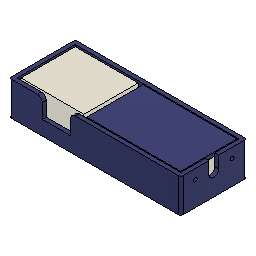
Breadboard Box Fusion (Autodesk Fusion 360 design; units mm, degrees)
Autodesk Fusion 360 part; units mm, degrees
sketch "Sketch1" plane through (0, 0, 0) normal (0, 1, 0) x (1, 0, 0)
  line L0 (0, 0) -> (165, 0)
  line L1 (165, 0) -> (165, -56)
  line L2 (165, -56) -> (0, -56)
  line L3 (0, -56) -> (0, 0)
  dimension "d1" = 165
  dimension "d2" = 56
  constraint horizontal L0
  constraint vertical L1
  constraint horizontal L2
  constraint vertical L3
  constraint coincident L0.start L3.end
  measures "d1" distance of L0.start L0.end
  measures "d2" distance of L0.start L2.end
extrude "Extrude1" add sketch "Sketch1" along normal blind 10 makes body 1
sketch "Sketch2" plane through (0, 10, 0) normal (0, 1, 0) x (-1, 0, 0)
  line L0 (0, 56) -> (-165, 56)
  line L1 (-165, 56) -> (-165, 0)
  line L2 (-165, 0) -> (0, 0)
  line L3 (0, 0) -> (0, 56)
  line L4 (0, 0) -> (-65, 0)
  line L5 (-65, 0) -> (-65, 56)
  line L6 (-65, 56) -> (0, 56)
  line L7 (0, 56) -> (0, 0)
  line L8 (-165, 15) -> (-115, 15)
  line L9 (-115, 15) -> (-115, 41)
  line L10 (-115, 41) -> (-165, 41)
  line L11 (-165, 41) -> (-165, 15)
  dimension "d5" = 65
  dimension "d8" = 15
  dimension "d9" = 15
  dimension "d10" = 50
  constraint horizontal L4
  constraint vertical L5
  constraint horizontal L6
  constraint vertical L7
  constraint coincident L2.end L3.start
  constraint horizontal L8
  constraint vertical L9
  constraint horizontal L10
  constraint vertical L11
  constraint coincident L1 L8.start
  measures "d5" distance of L2.end L4.end
  measures "d8" distance of L1.end L8.start
  measures "d9" distance of L0.end L10.end
  measures "d10" distance of L9 L11
extrude "Extrude2" add sketch "Sketch2" along normal blind 20 contours L0 L2 L3 L4 L5 L6 L7 bodies 1
extrude "Extrude3" add sketch "Sketch2" along normal blind 15 contours L1 L8 L9 L10 L11 bodies 1
sketch "Sketch3" plane through (0, 0, 0) normal (0, -1, 0) x (1, 0, 0)
  line L0 (165, 56) -> (0, 56)
  line L1 (0, 56) -> (0, 0)
  line L2 (0, 0) -> (165, 0)
  line L3 (165, 0) -> (165, 56)
  line L4 (-2, -2) -> (167, -2)
  line L5 (167, -2) -> (167, 58)
  line L6 (167, 58) -> (-2, 58)
  line L7 (-2, 58) -> (-2, -2)
  line L8 (-6, -6) -> (171, -6)
  line L9 (171, -6) -> (171, 62)
  line L10 (171, 62) -> (-6, 62)
  line L11 (-6, 62) -> (-6, -6)
  dimension "d13" = 2
  dimension "d14" = 6
extrude "Extrude4" add sketch "Sketch3" along normal blind 5 separate body contours L0 L1 L2 L3 | L4 L5 L6 L7 | L8 L9 L10 L11 makes body 2
extrude "Extrude5" add sketch "Sketch3" against normal blind 30 contours L8 L9 L10 L11 bodies 2
sketch "Sketch5" plane through (171, 0, 0) normal (1, 0, 0) x (0, 0, -1)
  line L0 (-62, 30) -> (-62, -5)
  line L1 (-62, -5) -> (6, -5)
  line L2 (6, -5) -> (6, 30)
  line L3 (6, 30) -> (-62, 30)
  line L4 (-28, 30) -> (-28, -5)
  line L5 (-28, 30) -> (-28, 17.5)
  arc A0 (-33, 17.5) -> (-23, 17.5) centre (-28, 17.5) ccw
  line L6 (-33, 17.5) -> (-33, 30)
  line L7 (-23, 17.5) -> (-23, 30)
  dimension "d19" = 12.5
  dimension "d20" = 5
  constraint midpoint L3 L4.start
  constraint midpoint L1 L4.end
  constraint perpendicular L3 L5
  constraint coincident L5.end A0.centre
  constraint coincident L3 L6.end
  constraint tangent A0 L6
  constraint perpendicular L3 L6
  constraint coincident L3 L7.end
  constraint tangent A0 L7
  constraint perpendicular L3 L7
  measures "d19" distance of L4.start L5.end
  measures "d20" radius of A0
extrude "Extrude6" cut sketch "Sketch5" against normal blind 4 contours L3 L4 L5 A0 L6 | L3 L4 L5 A0 L7 bodies 2
sketch "Sketch6" plane through (0, 30, 0) normal (0, 1, 0) x (-1, 0, 0)
  line L0 (-171, 33) -> (-167, 33)
  line L1 (-167, 33) -> (-167, 58)
  line L2 (-167, 58) -> (2, 58)
  line L3 (2, 58) -> (2, -2)
  line L4 (2, -2) -> (-167, -2)
  line L5 (-167, -2) -> (-167, 23)
  line L6 (-167, 23) -> (-171, 23)
  line L7 (-171, 23) -> (-171, -6)
  line L8 (-171, -6) -> (6, -6)
  line L9 (6, -6) -> (6, 62)
  line L10 (6, 62) -> (-171, 62)
  line L11 (-171, 62) -> (-171, 33)
  line L12 (0, 56) -> (-65, 56)
  line L13 (-65, 56) -> (-65, 0)
  line L14 (-65, 0) -> (0, 0)
  line L15 (0, 0) -> (0, 56)
  line L16 (-68, -2) -> (-68, 58)
  line L17 (-68, 58) -> (-167, 58)
  line L18 (-167, 58) -> (-167, -2)
  line L19 (-167, -2) -> (-68, -2)
  line L20 (-68, -2) -> (-68, 58)
  line L21 (-69, 57) -> (-166, 57)
  line L22 (-166, 57) -> (-166, -1)
  line L23 (-166, -1) -> (-69, -1)
  line L24 (-69, -1) -> (-69, 57)
  dimension "d23" = 3
  dimension "d35" = -1
  constraint coincident L4 L16.start
  constraint coincident L2 L16.end
  constraint perpendicular L2 L16
  constraint horizontal L17
  constraint vertical L18
  constraint horizontal L19
  constraint vertical L20
  constraint coincident L4.end L5.start
  measures "d23" distance of L13 L16
extrude "Extrude7" add sketch "Sketch6" against normal blind 4 separate body contours L21 L22 L23 L24 makes body 3
sketch "Sketch7" plane through (0, 0, -2) normal (0, 0, 1) x (1, 0, 0)
  line L0 (-2, 0) -> (167, 0)
  line L1 (167, 0) -> (167, 30)
  line L2 (167, 30) -> (-2, 30)
  line L3 (-2, 30) -> (-2, 0)
  line L4 (82.5, 30) -> (87.5, 30)
  line L5 (87.5, 30) -> (87.5, 18)
  line L6 (87.5, 18) -> (82.5, 18)
  line L7 (82.5, 18) -> (82.5, 30)
  line L8 (142.5, 30) -> (147.5, 30)
  line L9 (147.5, 30) -> (147.5, 18)
  line L10 (147.5, 18) -> (142.5, 18)
  line L11 (142.5, 18) -> (142.5, 30)
  line L12 (82.5, 28) -> (87.5, 28)
  line L13 (142.5, 28) -> (147.5, 28)
  dimension "d26" = 5
  dimension "d27" = 12
  dimension "d28" = 5
  dimension "d29" = 12
  dimension "d30" = 55
  dimension "d34" = 2
  constraint horizontal L4
  constraint vertical L5
  constraint horizontal L6
  constraint vertical L7
  constraint midpoint L2 L4.start
  constraint horizontal L8
  constraint vertical L9
  constraint horizontal L10
  constraint vertical L11
  constraint coincident L2 L8.start
  constraint coincident L7 L12.start
  constraint coincident L5 L12.end
  constraint perpendicular L5 L12
  constraint coincident L11 L13.start
  constraint coincident L9 L13.end
  constraint perpendicular L9 L13
  constraint collinear L12 L13
  measures "d26" distance of L4.start L4.end
  measures "d27" distance of L4.start L6.end
  measures "d28" distance of L8.start L8.end
  measures "d29" distance of L8.start L10.end
  measures "d30" distance of L5 L8.start
  measures "d34" distance of L4 L12
revolve "Revolve1" cut sketch "Sketch7" angle 10 about axis through (142.5, 28, -2) along (1, 0, 0) contours L5 L6 L7 L12 | L9 L10 L11 L13 bodies 2
ref_plane "WorkPlane1" through (82.5, 15, 28) normal (0, 0, 1) x (1, 0, 0)
mirror "Mirror1" about plane through (82.5, 15, 28) normal (0, 0, 1) of "Revolve1"
sketch "Sketch8" plane through (0, 26, 0) normal (0, -1, 0) x (1, 0, 0)
  line L0 (69, 57) -> (69, -1)
  line L1 (69, -1) -> (166, -1)
  line L2 (166, -1) -> (166, 57)
  line L3 (166, 57) -> (69, 57)
  line L4 (82.5, 58) -> (87.5, 58)
  line L5 (87.5, 58) -> (82.5, 58)
  line L6 (142.5, 58) -> (147.5, 58)
  line L7 (147.5, 58) -> (142.5, 58)
  line L8 (167, 58) -> (-2, 58)
  line L9 (-2, 58) -> (167, 58)
  line L10 (87.5, -2) -> (82.5, -2)
  line L11 (82.5, -2) -> (87.5, -2)
  line L12 (147.5, -2) -> (142.5, -2)
  line L13 (142.5, -2) -> (147.5, -2)
  line L14 (-2, -2) -> (167, -2)
  line L15 (167, -2) -> (-2, -2)
  line L16 (147.5, -1) -> (142.5, -1)
  line L17 (142.5, -1) -> (142.5, 2)
  line L18 (142.5, 2) -> (147.5, 2)
  line L19 (147.5, 2) -> (147.5, -1)
  line L20 (166, 28) -> (69, 28)
  line L21 (87.5, -1) -> (82.5, -1)
  line L22 (82.5, -1) -> (82.5, 2)
  line L23 (82.5, 2) -> (87.5, 2)
  line L24 (87.5, 2) -> (87.5, -1)
  line L25 (82.5, 54) -> (87.5, 54)
  line L26 (82.5, 57) -> (82.5, 54)
  line L27 (87.5, 54) -> (87.5, 57)
  line L28 (147.5, 54) -> (147.5, 57)
  line L29 (142.5, 54) -> (147.5, 54)
  line L30 (142.5, 57) -> (142.5, 54)
  dimension "d36" = 3
  dimension "d37" = 3
  constraint horizontal L16
  constraint vertical L17
  constraint horizontal L18
  constraint vertical L19
  constraint coincident L1 L16.start
  constraint midpoint L2 L20.start
  constraint midpoint L0 L20.end
  constraint horizontal L21
  constraint vertical L22
  constraint horizontal L23
  constraint vertical L24
  constraint coincident L1 L21.start
  constraint collinear L10.end L21.end L22.end
  constraint vertical L10.start L21.start
  constraint vertical L12.end L16.end
  constraint vertical L12.start L16.start
  constraint symmetric L16.start L20 L28.end
  constraint symmetric L16.end L20 L30.start
  constraint symmetric L17.end L20 L29.start
  constraint symmetric L18.end L20 L28.start
  constraint symmetric L20 L21.start L27.end
  constraint symmetric L20 L21.end L26.start
  constraint symmetric L20 L22.end L25.start
  constraint symmetric L20 L23.end L25.end
  measures "d36" distance of L16.start L18.end
  measures "d37" distance of L21.start L23.end
extrude "Extrude8" add sketch "Sketch8" along normal blind 7.5 contours L3 L25 L26 L27 | L1 L21 L22 L23 L24 | L3 L28 L29 L30 | L1 L16 L17 L18 L19 bodies 3
sketch "Sketch9" plane through (0, 0, 57) normal (0, 0, 1) x (1, 0, 0)
  line L0 (166, 30) -> (69, 30)
  line L1 (69, 30) -> (69, 26)
  line L2 (69, 26) -> (82.5, 26)
  line L3 (82.5, 26) -> (82.5, 18.5)
  line L4 (82.5, 18.5) -> (87.5, 18.5)
  line L5 (87.5, 18.5) -> (87.5, 26)
  line L6 (87.5, 26) -> (142.5, 26)
  line L7 (142.5, 26) -> (142.5, 18.5)
  line L8 (142.5, 18.5) -> (147.5, 18.5)
  line L9 (147.5, 18.5) -> (147.5, 26)
  line L10 (147.5, 26) -> (166, 26)
  line L11 (166, 26) -> (166, 30)
  line L12 (82.5, 26) -> (87.5, 26)
  line L13 (87.5, 26) -> (87.5, 18.5)
  line L14 (87.5, 18.5) -> (82.5, 18.5)
  line L15 (82.5, 18.5) -> (82.5, 26)
  line L16 (142.5, 18.5) -> (147.5, 18.5)
  line L17 (147.5, 18.5) -> (147.5, 26)
  line L18 (147.5, 26) -> (142.5, 26)
  line L19 (142.5, 26) -> (142.5, 18.5)
  constraint horizontal L12
  constraint vertical L13
  constraint horizontal L14
  constraint vertical L15
  constraint coincident L4.end L5.start
  constraint coincident L2.end L3.start
  constraint horizontal L16
  constraint vertical L17
  constraint horizontal L18
  constraint vertical L19
  constraint coincident L9.end L10.start
  constraint coincident L7.end L8.start
revolve "Revolve2" add sketch "Sketch9" angle 15 about axis through (82.5, 26, 57) along (-1, 0, 0) contours L7 L8 L9 L16 L17 L18 L19 | L3 L4 L5 L12 L13 L14 L15 bodies 3
sketch "Sketch10" plane through (0, 0, -1) normal (0, 0, -1) x (-1, 0, 0)
  line L0 (-69, 30) -> (-166, 30)
  line L1 (-166, 30) -> (-166, 26)
  line L2 (-166, 26) -> (-147.5, 26)
  line L3 (-147.5, 26) -> (-147.5, 18.5)
  line L4 (-147.5, 18.5) -> (-142.5, 18.5)
  line L5 (-142.5, 18.5) -> (-142.5, 26)
  line L6 (-142.5, 26) -> (-87.5, 26)
  line L7 (-87.5, 26) -> (-87.5, 18.5)
  line L8 (-87.5, 18.5) -> (-82.5, 18.5)
  line L9 (-82.5, 18.5) -> (-82.5, 26)
  line L10 (-82.5, 26) -> (-69, 26)
  line L11 (-69, 26) -> (-69, 30)
  line L12 (-87.5, 26) -> (-82.5, 26)
  line L13 (-142.5, 26) -> (-147.5, 26)
  constraint coincident L6.end L7.start
  constraint coincident L9.end L10.start
  constraint coincident L5.end L6.start
  constraint coincident L2.end L3.start
revolve "Revolve3" add sketch "Sketch10" angle 15 about axis through (87.5, 26, -1) along (1, 0, 0) contours L7 L8 L9 L12 | L3 L4 L5 L13 bodies 3
fillet "Fillet1" radius 1.5 4 edges at (145, 18.7556, 58.9411) (85, 18.7556, 58.9411) (85, 18.7556, -2.9411) (145, 18.7556, -2.9411) on bodies 3
sketch "Sketch11" plane through (171, 0, 0) normal (1, 0, 0) x (0, 0, -1)
  line L0 (-33, 17.5) -> (-33, 30)
  line L1 (-33, 30) -> (-62, 30)
  line L2 (-62, 30) -> (-62, -5)
  line L3 (-62, -5) -> (6, -5)
  line L4 (6, -5) -> (6, 30)
  line L5 (6, 30) -> (-23, 30)
  line L6 (-23, 30) -> (-23, 17.5)
  arc A0 (-33, 17.5) -> (-23, 17.5) centre (-28, 17.5) ccw
  circle A1 centre (-47, 20) radius 2
  circle A2 centre (-9, 20) radius 2
  dimension "d44" = 4
  dimension "d45" = 4
  dimension "d46" = 15
  dimension "d47" = 15
  dimension "d48" = 10
  constraint horizontal A1.centre A2.centre
  measures "d44" diameter of A1
  measures "d45" diameter of A2
  measures "d46" distance of L2 A1.centre
  measures "d47" distance of L4 A2.centre
  measures "d48" distance of L1 A1.centre
extrude "Extrude9" cut sketch "Sketch11" against normal blind 5 contours A1 | A2 bodies 2
sketch "Sketch12" plane through (0, 0, 62) normal (0, 0, 1) x (1, 0, 0)
  line L0 (-6, 30) -> (-6, -5)
  line L1 (-6, -5) -> (171, -5)
  line L2 (171, -5) -> (171, 30)
  line L3 (171, 30) -> (-6, 30)
  line L4 (28, 30) -> (57, 30)
  line L5 (57, 30) -> (57, 10)
  line L6 (57, 10) -> (28, 10)
  line L7 (28, 10) -> (28, 30)
  line L8 (115, 10) -> (165, 10)
  line L9 (165, 10) -> (65, 10)
  line L10 (65, 10) -> (165, 10)
  line L11 (165, 10) -> (115, 10)
  dimension "d51" = 34
  dimension "d52" = 63
  constraint horizontal L4
  constraint vertical L5
  constraint horizontal L6
  constraint vertical L7
  constraint coincident L3 L4.start
  constraint collinear L6 L9
  measures "d51" distance of L0 L7
  measures "d52" distance of L0 L5
extrude "Extrude10" cut sketch "Sketch12" against normal blind 5 contours L3 L4 L5 L6 L7 bodies 2
fillet "Fillet2" radius 5 2 edges at (57, 30, 60) (28, 30, 60) on bodies 2
fillet "Fillet3" radius 2.5 4 edges at (-6, 12.5, 62) (-6, 12.5, -6) (171, 12.5, -6) (171, 12.5, 62) on bodies 2
equation "d45 = d44"
equation "d47 = d46"
named bodies: "Breadboard+Sensors+Feather", "Main Case Body", "Top Cover"
